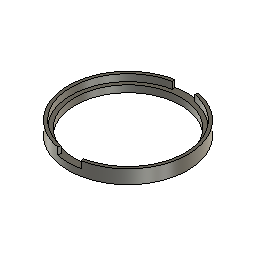
nato_socket_seal (Autodesk Fusion 360 design; units mm, degrees)
part number: 2026-08-05-17-22-02-167
Autodesk Fusion 360 part; units mm, degrees
sketch "Sketch1" plane through (0, 0, 0) normal (0, 0, 1) x (1, 0, 0)
  circle A0 centre (0, 0) radius 27
  circle A1 centre (0, 0) radius 29
  dimension "d1" = 54
  dimension "d2" = 58
  constraint coincident A0.centre A1.centre
  measures "d1" diameter of A0
  measures "d2" diameter of A1
extrude "Extrude1" add sketch "Sketch1" along normal blind 3.5
sketch "Sketch2" plane through (0, 0, 0) normal (0, 0, -1) x (1, 0, 0)
  circle A0 centre (0, 0) radius 27
  circle A1 centre (0, 0) radius 29
  circle A2 centre (0, 0) radius 30.5
  dimension "d5" = 61
  constraint coincident A0.centre A1.centre
  measures "d5" diameter of A2
extrude "Extrude2" add sketch "Sketch2" against normal blind 7 contours A2
sketch "Sketch3" plane through (0, 0, 7) normal (0, 0, 1) x (-1, 0, 0)
  circle A0 centre (0, 0) radius 29
  circle A1 centre (0, 0) radius 30.5
  line L0 (0, 29.5) -> (-6, 29.5) construction
  line L1 (0, 26) -> (0, 34.5) construction
  line L2 (0, 29.5) -> (6, 29.5) construction
  line L3 (5.7478, 28.4247) -> (6.0905, 29.8857)
  line L4 (-5.7478, 28.4247) -> (-6.0905, 29.8857)
  line L5 (-6, 0) -> (15.5156, 0) construction
  line L6 (5.7478, -28.4247) -> (6.0905, -29.8857)
  line L7 (-5.7478, -28.4247) -> (-6.0905, -29.8857)
  dimension "d8" = 6
  constraint horizontal L0
  constraint vertical L1
  constraint symmetric L0.start L1 L2.start
  constraint symmetric L0.end L1 L2.end
  constraint coincident A0 L3.start
  constraint coincident A1 L3.end
  constraint coincident L2.end L3
  constraint symmetric L1 L3.start L4.start
  constraint symmetric L1 L3.end L4.end
  constraint horizontal L5
  constraint symmetric L3.start L5 L6.start
  constraint symmetric L3.end L5 L6.end
  constraint symmetric L4.start L5 L7.start
  constraint symmetric L4.end L5 L7.end
  measures "d8" distance of L0.start L0.end
extrude "Extrude3" cut sketch "Sketch3" against normal blind 3.5 contours A0 A1 L3 L4
extrude "Extrude4" cut sketch "Sketch3" against normal blind 3.5 contours A0 A1 L6 L7
